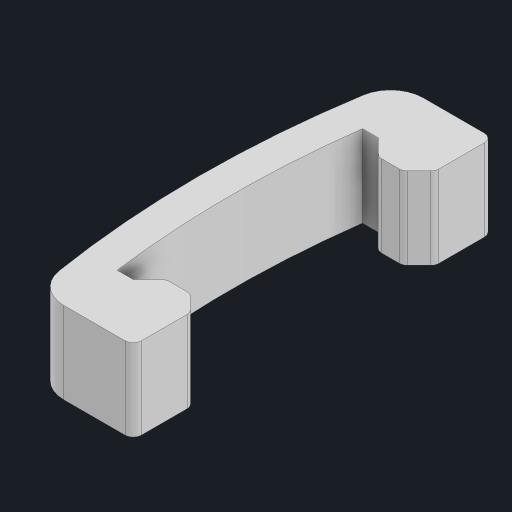
# Autodesk Inventor part: Mounting Clip
Saved by Autodesk Inventor 2023.1 (Build 271208000, 208)
## iProperties
Created: 2023-02-28
Part Number: Mounting Clip
Material: Generic
Document SubType Name: Modeling
Designer: Jarrett
Density: 1 g/cm^3
Appearance: Default
Author: Jarrett
Autodesk Inventor part; units mm, degrees
ref_plane "YZ Plane" through (0, 0, 0) normal (1, 0, 0) x (0, 1, 0)
ref_plane "XZ Plane" through (0, 0, 0) normal (0, 1, 0) x (-1, 0, 0)
ref_plane "XY Plane" through (0, 0, 0) normal (0, 0, 1) x (1, 0, 0)
sketch "Sketch1" plane through (0, 0, 0) normal (0, 1, 0) x (-1, 0, 0)
  circle A0 centre (0, 0) radius 2.15
  line L0 (-10, 10) -> (10, 10)
  line L1 (10, 10) -> (10, -10)
  line L2 (10, -10) -> (-10, -10)
  line L3 (-10, -10) -> (-10, 10)
  line L4 (-10, 10) -> (10, -10) construction
  line L5 (10, 10) -> (-10, -10) construction
  line L6 (10, -2.5) -> (8.5267, -2.5)
  line L7 (8.5267, -2.5) -> (8.5267, -4.8839)
  line L8 (7.0482, -5.4963) -> (3.6, -2.0481)
  line L9 (3.6, -2.0481) -> (3.6, 2.0481)
  line L10 (3.6, 2.0481) -> (7.0482, 5.4963)
  line L11 (8.5267, 4.8839) -> (8.5267, 2.5)
  line L12 (8.5267, 2.5) -> (10, 2.5)
  line L13 (0, 0) -> (10, 0) construction
  arc A1 (8.5267, 4.8839) -> (7.0482, 5.4963) centre (7.6606, 4.8839) ccw
  arc A2 (7.0482, -5.4963) -> (8.5267, -4.8839) centre (7.6606, -4.8839) ccw
  line L14 (8.5267, -24.8839) -> (8.5267, -22.5)
  arc A3 (7.0482, -25.4963) -> (8.5267, -24.8839) centre (7.6606, -24.8839) ccw
  line L15 (3.6, -22.0481) -> (7.0482, -25.4963)
  line L16 (3.6, -17.9519) -> (3.6, -22.0481)
  arc A4 (8.5267, -15.1161) -> (7.0482, -14.5037) centre (7.6606, -15.1161) ccw
  line L17 (7.0482, -14.5037) -> (3.6, -17.9519)
  line L18 (10, -30) -> (10, -10)
  line L19 (8.5267, -22.5) -> (10, -22.5)
  line L20 (10, -17.5) -> (8.5267, -17.5)
  line L21 (8.5267, -17.5) -> (8.5267, -15.1161)
  arc A5 (10, -17.5) -> (10.5, -10) centre (-46, -10) ccw
  arc A6 (11.4565, -21) -> (12.5, -10) centre (-46, -10) ccw
  line L22 (11.4565, -21) -> (5.5267, -21)
  line L23 (5.5267, -21) -> (5.5267, -17.5)
  line L24 (5.5267, -17.5) -> (6.5267, -16.5)
  line L25 (6.5267, -16.5) -> (8.0267, -16.5)
  line L26 (8.0267, -16.5) -> (9.0267, -17.5)
  line L27 (9.0267, -17.5) -> (10, -17.5)
  line L28 (10, -10) -> (12.5, -10)
  point P0 (8.5267, -6.9748)
  point P1 (8.5267, 6.9748)
  point P2 (3.6, 0)
  point P3 (8.5267, -3.692)
  dimension "d0" = 4.3
  dimension "d1" = 20
  dimension "d2" = 20
  dimension "d3" = 5
  dimension "d4" = 6.4
  dimension "d5" = 11.5
  dimension "d6" = 2
  dimension "d8" = 1
  dimension "d9" = 45
  dimension "d10" = 45
  dimension "d11" = 3
  dimension "d12" = 1.5
  dimension "d13" = 0.5
  dimension "d14" = 0.5
  constraints: 58 end point, 14 point on line, 13 symmetric about line, 12 point on circle, 7 centre point, 6 parallel, 5 midpoint, 5 perpendicular, 4 horizontal, 4 tangent, 2 collinear, 2 vertical, 1 coincident, 1 equal radius, 1 line through centre, 3 other
  measures "d0" diameter of A0
  measures "d1" distance of L2.start L2.end
  measures "d2" distance of L0.end L2.start
  measures "d3" distance between parallel lines of L6 L12
  measures "d4" distance between parallel lines of L9 L1
  measures "d6" radial gap between concentric circles of A6 A5
  measures "d8" distance between parallel lines of L25 L20
  measures "d9" angle of L25 L26
  measures "d10" angle of L25 L24
  measures "d11" distance between parallel lines of L21 L23
  measures "d12" distance between parallel lines of L22 L19
  measures "d13" distance from line of L26.end L21
  measures "d14" distance from line of L18 A5.end
extrude "Extrusion1" add sketch "Sketch1" along normal blind 5 contours A5 L28 A6 L22 L18 | L18 L22 L23 L24 L25 L26 L21 L20 | L20 L21 L26
mirror "Mirror1" about plane through (-12.5, 0, -10) normal (0, 0, 1) of "Extrusion1"
fillet "Fillet1" radius 2 2 edges at (-11.4565, 2.5, 1) (-11.4565, 2.5, -21)
fillet "Fillet2" radius 0.5 8 edges at (-8.0267, 2.5, -16.5) (-6.5267, 2.5, -16.5) (-5.5267, 2.5, -17.5) (-5.5267, 2.5, -21) (-5.5267, 2.5, 1) (-5.5267, 2.5, -2.5) (-8.0267, 2.5, -3.5) (-6.5267, 2.5, -3.5)
body "Solid1"
